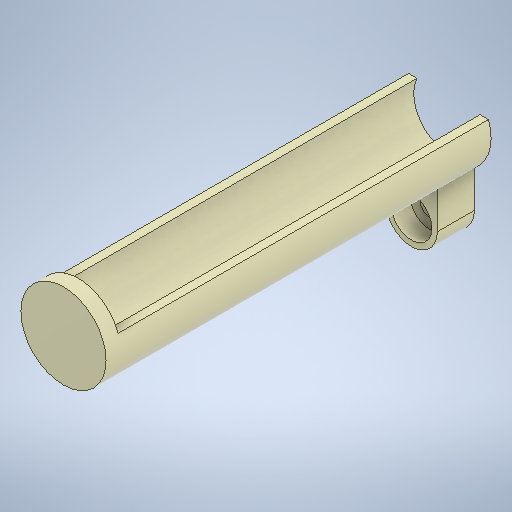
# Autodesk Inventor part: pen_limiter
Saved by Autodesk Inventor 2025.1 (Build 291241000, 241)
## iProperties
Created: 2024-08-25
Part Number: pen_limiter
Material: Polypropylene
Document SubType Name: Modeling
Designer: pedro
Density: 0.899 g/cm^3
Appearance: Smooth - Ash
Author: pedro
Autodesk Inventor part; units mm, degrees
ref_plane "YZ Plane" through (0, 0, 0) normal (1, 0, 0) x (0, 1, 0)
ref_plane "XZ Plane" through (0, 0, 0) normal (0, 1, 0) x (-1, 0, 0)
ref_plane "XY Plane" through (0, 0, 0) normal (0, 0, 1) x (1, 0, 0)
sketch "Sketch1" plane through (0, 0, 0) normal (0, 0, 1) x (1, 0, 0)
  arc A0 (-4.2532, 2) -> (4.2532, 2) centre (0, 0) ccw
  arc A1 (-5.391, 2) -> (5.391, 2) centre (0, 0) ccw
  line L0 (-5.391, 2) -> (-4.2532, 2)
  line L1 (4.2532, 2) -> (5.391, 2)
  dimension "d0" = 9.4
  dimension "d1" = 11.5
  constraints: 4 end point, 4 point on circle, 2 centre point, 2 coincident, 2 horizontal
  measures "d0" diameter of A0
  measures "d1" diameter of A1
extrude "Extrusion1" add sketch "Sketch1" along normal blind 50
sketch "Sketch2" plane through (0, 0, 50) normal (0, 0, 1) x (1, 0, 0)
  circle A0 centre (0, 0) radius 5.75
  constraints: 1 centre point
extrude "Extrusion2" add sketch "Sketch2" along normal blind 2
sketch "Sketch3" plane through (0, 0, 0) normal (0, 0, -1) x (-1, 0, 0)
  arc A0 (-5.391, 2) -> (5.391, 2) centre (0, 0) ccw projected
  arc A1 (-3.5, -9.5621) -> (3.5, -9.5621) centre (0, -9.5621) ccw
  line L0 (3.5, -9.5621) -> (3.5, -4.5621)
  line L1 (-3.5, -9.5621) -> (-3.5, -4.5621)
  dimension "d7" = 7
  dimension "d9" = 5
  constraints: 4 end point, 4 point on circle, 2 vertical, 1 centre point, 1 tangent
  measures "d7" diameter of A1
  measures "d9" distance of L0.start L0.end
extrude "Extrusion3" add sketch "Sketch3" against normal blind 5
sketch "Sketch4" plane through (0, 0, 0) normal (0, 0, -1) x (-1, 0, 0)
  arc A0 (-3.5, -9.5621) -> (3.5, -9.5621) centre (0, -9.5621) ccw projected
  circle A1 centre (0, -9.5621) radius 1.35
  point P0 (0, 0)
  dimension "d12" = 2.7
  constraints: 1 centre point, 1 coincident
  measures "d12" diameter of A1
extrude "Extrusion4" cut sketch "Sketch4" against normal through all
sketch "Sketch5" plane through (0, 0, 5) normal (0, 0, 1) x (1, 0, 0)
  circle A0 centre (0, -9.5621) radius 1.35 projected
  circle A1 centre (0, -9.5621) radius 2.75
  point P0 (0, 0)
  dimension "d15" = 5.5
  constraints: 1 centre point, 1 coincident
  measures "d15" diameter of A1
extrude "Extrusion5" cut sketch "Sketch5" against normal blind 2.5
body "Solid1"
